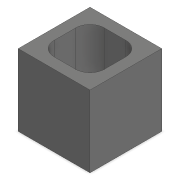
# Autodesk Inventor part: adocreto
Saved by Autodesk Inventor 2020 (Build 240168000, 168)
## iProperties
Created: 2022-05-05
Part Number: adocreto
Material: Generic
Document SubType Name: Modeling
Designer: leo
Density: 1 g/cm^3
Appearance: Gray
Author: leo
Autodesk Inventor part; units mm, degrees
ref_plane "YZ Plane" through (0, 0, 0) normal (1, 0, 0) x (0, 1, 0)
ref_plane "XZ Plane" through (0, 0, 0) normal (0, 1, 0) x (-1, 0, 0)
ref_plane "XY Plane" through (0, 0, 0) normal (0, 0, 1) x (1, 0, 0)
sketch "Sketch1" plane through (0, 0, 0) normal (0, 1, 0) x (-1, 0, 0)
  line L0 (100, 100) -> (-100, 100)
  line L1 (-100, 100) -> (-100, -100)
  line L2 (-100, -100) -> (100, -100)
  line L3 (100, -100) -> (100, 100)
  line L4 (30, 70) -> (-30, 70)
  line L5 (-70, 30) -> (-70, -30)
  line L6 (-30, -70) -> (30, -70)
  line L7 (70, -30) -> (70, 30)
  arc A0 (30, -70) -> (70, -30) centre (30, -30) ccw
  arc A1 (-70, -30) -> (-30, -70) centre (-30, -30) ccw
  arc A2 (-30, 70) -> (-70, 30) centre (-30, 30) ccw
  arc A3 (70, 30) -> (30, 70) centre (30, 30) ccw
  point P0 (0, 0)
  point P1 (100, 0)
  point P2 (0, -100)
  dimension "d0" = 200
  dimension "d1" = 30
  dimension "d2" = 40
  constraints: 16 end point, 8 point on circle, 8 tangent, 4 centre point, 4 parallel, 3 equal radius, 3 perpendicular, 2 midpoint, 1 horizontal, 1 horizontal alignment, 1 vertical alignment, 3 other
  measures "d0" distance of L2.end L0.start
  measures "d1" distance between parallel lines of L2 L6
  measures "d2" radius of A0
extrude "Extrusion1" add sketch "Sketch1" along normal blind 200
body "Solid1"
